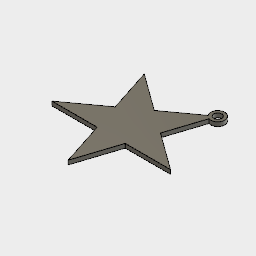
五角星挂件 v1 (Autodesk Fusion 360 design; units mm, degrees)
Autodesk Fusion 360 part; units mm, degrees
note: some values were not read from the file. Set by a fixed rule: which sketch regions a step uses.
sketch "草图1" plane through (0, 0, 0) normal (0, 1, 0) x (1, 0, 0)
  line L0 (-52.5144, 0) -> (-26.2572, -80.8114)
  line L1 (0, 0) -> (-26.2572, -80.8114)
  line L2 (0, 0) -> (-68.7423, -49.9442)
  line L3 (-68.7423, -49.9442) -> (16.2279, -49.9442)
  line L4 (16.2279, -49.9442) -> (-52.5144, 0)
  circle A0 centre (0, 0) radius 5
  circle A1 centre (0, 0) radius 2.8284
  point P0 (-26.2572, -36.14)
extrude "拉伸1" add sketch "草图1" along normal blind 3 contours L0 L2 L4 | L0 L1 L2 L3 L4 | L0 L2 L3 | L1 L2 L4 A0 | L0 L1 L3 | L1 L2 A0 A1 | L1 L2 A0 A1 | L1 L3 L4
